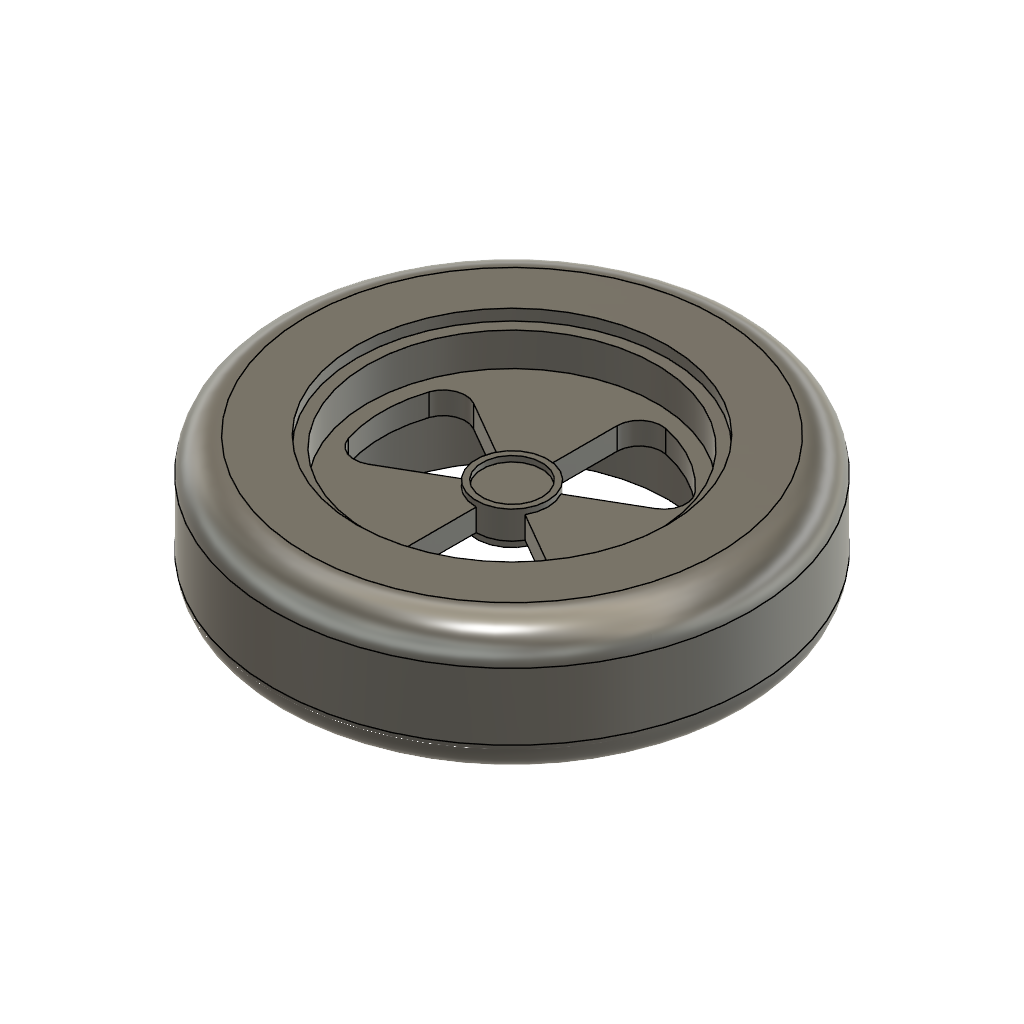
tyre (Autodesk Fusion 360 design; units mm, degrees)
part number: 2026-10-04-21-21-09-856
Autodesk Fusion 360 part; units mm, degrees
sketch "Sketch1" plane through (0, 0, 0) normal (0, 1, 0) x (1, 0, 0)
  circle A0 centre (0, 0) radius 21.5
  circle A1 centre (0, 0) radius 14
  circle A2 centre (0, 0) radius 13
  dimension "d1" = 43
  dimension "d2" = 28
  dimension "d3" = 26
  constraint coincident A0.centre A1.centre
  constraint concentric A0 A1
  constraint concentric A0 A2
  measures "d1" diameter of A0
  measures "d2" diameter of A1
  measures "d3" diameter of A2
extrude "Extrude1" add sketch "Sketch1" along normal mid plane 12 contours A0
extrude "Extrude2" add sketch "Sketch1" along normal blind 5 contours A1
extrude "Extrude3" add sketch "Sketch1" along normal blind 2 contours A2
fillet "Fillet1" radius 3 2 edges at (-20.045, 6, 7.7747) (-20.045, -6, -7.7747)
sketch "Sketch2" plane through (0, 2, 0) normal (0, 1, 0) x (-1, 0, 0)
  circle A0 centre (0, 0) radius 13
  line L0 (0, 0) -> (0, -13)
  line L1 (0, 0) -> (-11.253, 6.5092)
  line L2 (0, 0) -> (11.253, 6.5092)
  line L3 (0, 0) -> (-11.253, -6.5092)
  line L4 (0, 0) -> (0, 13)
  line L5 (11.253, -6.5092) -> (-11.253, 6.5092)
  circle A1 centre (0, 0) radius 11.6863
  constraint coincident A0.centre L0.start
  constraint coincident A0 L0.end
  constraint vertical L0
  constraint coincident A0 L1.end
  constraint coincident A0 L2.end
  constraint coincident A0 L3.end
  constraint parallel L2 L3
  constraint coincident A0 L4.end
  constraint vertical L4
  constraint midpoint A0.centre L5
extrude "Extrude4" cut sketch "Sketch2" against normal blind 17 contours L2 L5 A1 | L1 L4 L5 A1 | L0 L3 A1
fillet "Fillet2" radius 2 6 edges at (0, 1, -11.6863) (10.1158, 1, 5.8514) (0, 1, 11.6863) (-10.1158, 1, 5.8514) (10.1158, 1, -5.8514) (-10.1158, 1, -5.8514)
sketch "Sketch3" plane through (0, 2, 0) normal (0, 1, 0) x (-1, 0, 0)
  arc A0 (11.106, -3.6366) -> (11.106, 3.6366) centre (0, 0) ccw
  arc A1 (8.2039, -4.7455) -> (11.106, -3.6366) centre (9.2053, -3.0142) ccw
  line L0 (8.2039, -4.7455) -> (0, 0)
  line L1 (0, 0) -> (0, -9.4775)
  arc A2 (-2.413, -11.4344) -> (0, -9.4775) centre (-2, -9.4775) ccw
  arc A3 (-8.6897, -7.814) -> (-2.413, -11.4344) centre (0, 0) ccw
  arc A4 (-8.2039, -4.7455) -> (-8.6897, -7.814) centre (-7.2025, -6.4767) ccw
  line L2 (-8.2039, -4.7455) -> (0, 0)
  line L3 (0, 0) -> (-8.2039, 4.7455)
  arc A5 (-8.6897, 7.814) -> (-8.2039, 4.7455) centre (-7.2025, 6.4767) ccw
  arc A6 (-2.413, 11.4344) -> (-8.6897, 7.814) centre (0, 0) ccw
  arc A7 (0, 9.4775) -> (-2.413, 11.4344) centre (-2, 9.4775) ccw
  line L4 (0, 9.4775) -> (0, 0)
  line L5 (0, 0) -> (8.2039, 4.7455)
  arc A8 (11.106, 3.6366) -> (8.2039, 4.7455) centre (9.2053, 3.0142) ccw
  circle A9 centre (0, 0) radius 13
  circle A10 centre (0, 0) radius 3.2281
  circle A11 centre (0, 0) radius 2.7011
  constraint coincident A0.centre L0.end
  constraint concentric A10 A11
extrude "Extrude5" add sketch "Sketch3" against normal blind 2 contours L0 L1 A10 A11 | L0 L5 A10 A11 | L4 L5 A10 A11 | L0 L1 A11 | L0 L5 A11 | L1 L2 A10 A11 | L4 L5 A11 | L3 L4 A10 A11 | L1 L2 A11 | L2 L3 A11 | L3 L4 A11 | L2 L3 A10 A11
sketch "Sketch4" plane through (0, 2, 0) normal (0, 1, 0) x (-1, 0, 0)
  line L0 (0, -3.2281) -> (0, -9.4775)
  arc A0 (-2.413, -11.4344) -> (0, -9.4775) centre (-2, -9.4775) ccw
  arc A1 (-8.6897, -7.814) -> (-2.413, -11.4344) centre (0, 0) ccw
  arc A2 (-8.2039, -4.7455) -> (-8.6897, -7.814) centre (-7.2025, -6.4767) ccw
  line L1 (-8.2039, -4.7455) -> (-2.7943, -1.6163)
  arc A3 (-2.7943, -1.6163) -> (0, -3.2281) centre (0, 0) ccw
  line L2 (-2.7943, 1.6163) -> (-8.2039, 4.7455)
  arc A4 (-8.6897, 7.814) -> (-8.2039, 4.7455) centre (-7.2025, 6.4767) ccw
  arc A5 (-2.413, 11.4344) -> (-8.6897, 7.814) centre (0, 0) ccw
  arc A6 (0, 9.4775) -> (-2.413, 11.4344) centre (-2, 9.4775) ccw
  line L3 (0, 9.4775) -> (0, 3.2281)
  arc A7 (0, 3.2281) -> (-2.7943, 1.6163) centre (0, 0) ccw
  arc A8 (2.7943, -1.6163) -> (2.7943, 1.6163) centre (0, 0) ccw
  line L4 (2.7943, 1.6163) -> (8.2039, 4.7455)
  arc A9 (11.106, 3.6366) -> (8.2039, 4.7455) centre (9.2053, 3.0142) ccw
  arc A10 (11.106, -3.6366) -> (11.106, 3.6366) centre (0, 0) ccw
  arc A11 (8.2039, -4.7455) -> (11.106, -3.6366) centre (9.2053, -3.0142) ccw
  line L5 (8.2039, -4.7455) -> (2.7943, -1.6163)
  circle A12 centre (0, 0) radius 13
  circle A13 centre (0, 0) radius 3.25
  circle A14 centre (0, 0) radius 2.7033
  circle A15 centre (0, 0) radius 2.7011
  circle A16 centre (0, 0) radius 3.2281
  circle A17 centre (0, 0) radius 3.25
  dimension "d18" = 6.5
  constraint coincident A1.centre A3.centre
  constraint concentric A13 A14
  measures "d18" diameter of A13
extrude "Extrude6" add sketch "Sketch3" along normal blind 0.5 contours L0 L1 A10 A11 | L0 L5 A10 A11 | L4 L5 A10 A11 | L1 L2 A10 A11 | L3 L4 A10 A11 | L2 L3 A10 A11
sketch "Sketch5" plane through (0, 0, 0) normal (0, 1, 0) x (1, 0, 0)
  circle A0 centre (0, 0) radius 3.2294
  circle A1 centre (0, 0) radius 2.6936
  constraint coincident A0.centre A1.centre
  constraint concentric A0 A1
extrude "Extrude7" add sketch "Sketch5" against normal blind 0.5
